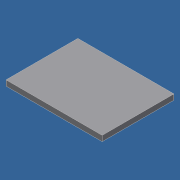
# Autodesk Inventor part: P1704_010_startSelectPCB
Saved by Autodesk Inventor 2019 (Build 230136000, 136)
## iProperties
Created: 2019-05-07
Part Number: P1704_010_startSelectPCB
Project: Nom Projet
Material: .
Description: Nom pièce
Document SubType Name: Modeling
Designer: Joan.MAILLARD
Authority: brut Ø
Density: 0.001 g/cm^3
Appearance: Par défaut
Material number: ---
Author: Joan.MAILLARD
Autodesk Inventor part; units mm, degrees
ref_plane "Plan YZ" through (0, 0, 0) normal (1, 0, 0) x (0, 1, 0)
ref_plane "Plan XZ" through (0, 0, 0) normal (0, 1, 0) x (-1, 0, 0)
ref_plane "Plan XY" through (0, 0, 0) normal (0, 0, 1) x (1, 0, 0)
sketch "Esquisse1" plane through (0, 0, 0) normal (0, 0, 1) x (1, 0, 0)
  line L0 (-17.675, -13.2) -> (17.675, -13.2)
  line L1 (17.675, -13.2) -> (17.675, 13.2)
  line L2 (17.675, 13.2) -> (-17.675, 13.2)
  line L3 (-17.675, 13.2) -> (-17.675, -13.2)
  line L4 (-17.675, -13.2) -> (17.675, 13.2) construction
  line L5 (17.675, -13.2) -> (-17.675, 13.2) construction
  point P0 (0, 0)
  dimension "d0" = 35.35
  dimension "d1" = 26.4
  constraints: 12 end point, 2 midpoint, 2 parallel, 1 horizontal, 1 perpendicular
  measures "d0" distance of L1.end L2.end
  measures "d1" distance of L0.end L1.end
extrude "Extrusion1" add sketch "Esquisse1" along normal blind 2
